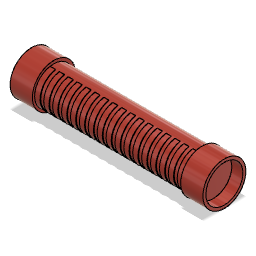
T-Stick (Autodesk Fusion 360 design; units mm, degrees)
Autodesk Fusion 360 part; units mm, degrees
note: some values were not read from the file. Chosen so that the rebuilt part matches the saved one: which bodies a step acts on.
sketch "Sketch1" plane through (0, 0, 0) normal (0, 0, 1) x (1, 0, 0)
  circle A0 centre (0, 0) radius 25
  circle A1 centre (0, 0) radius 29
  dimension "d3" = 50
  dimension "d4" = 4
  constraint coincident A0.centre A1.centre
  measures "d3" diameter of A0
extrude "Extrude1" add sketch "Sketch1" along normal blind 200 contours A0 makes body 1
extrude "Extrude2" add sketch "Sketch1" against normal blind 30 separate body makes body 2
extrude "Extrude3" add sketch "Sketch1" against normal blind 15 contours A0 bodies 1 2
sketch "Sketch2" plane through (0, 0, 200) normal (0, 0, 1) x (1, 0, 0)
  circle A0 centre (0, 0) radius 25
  circle A1 centre (0, 0) radius 29
  dimension "d9" = 4
extrude "Extrude4" add sketch "Sketch2" along normal blind 15 contours A0 bodies 1
extrude "Extrude5" add sketch "Sketch2" along normal blind 30 bodies 1
copy_body "CopyPasteBodies1" bodies 1 makes body 3
move_body "Move1" bodies 3 to x (1, 0, 0) y (0, 1, 0) z (0, 0, 1) at (0, 1, 0)
split "Split1" by plane through (0, 1, 200) normal (0, 0, -1) bodies 3 makes body 4 at (24.9689, -0.2461, 133.3333)
delete_body "RemoveBody1" bodies 3
split "Split2" by plane through (0, 1, 0) normal (0, 0, 1) bodies 4 makes body 5 at (24.9689, -0.2461, 133.3333)
delete_body "RemoveBody2" bodies 4
ref_plane "WorkPlane1" through (0, 26, 104.4776) normal (0, 1, 0) x (1, 0, 0)
sketch "Sketch3" plane through (0, 26, 104.4776) normal (0, 1, 0) x (1, 0, 0)
  line L0 (-26.9693, 97.1014) -> (24.8744, 97.1014)
  line L1 (24.8744, 97.1014) -> (24.8744, 92.1014)
  line L2 (24.8744, 92.1014) -> (-26.9693, 92.1014)
  line L3 (-26.9693, 92.1014) -> (-26.9693, 97.1014)
  line L4 (24.8744, 85.1014) -> (24.8744, 80.1014)
  line L5 (-26.9693, 80.1014) -> (-26.9693, 85.1014)
  line L6 (24.8744, 80.1014) -> (-26.9693, 80.1014)
  line L7 (-26.9693, 85.1014) -> (24.8744, 85.1014)
  line L8 (24.8744, 73.1014) -> (24.8744, 68.1014)
  line L9 (-26.9693, 68.1014) -> (-26.9693, 73.1014)
  line L10 (24.8744, 68.1014) -> (-26.9693, 68.1014)
  line L11 (-26.9693, 73.1014) -> (24.8744, 73.1014)
  line L12 (24.8744, 61.1014) -> (24.8744, 56.1014)
  line L13 (-26.9693, 56.1014) -> (-26.9693, 61.1014)
  line L14 (24.8744, 56.1014) -> (-26.9693, 56.1014)
  line L15 (-26.9693, 61.1014) -> (24.8744, 61.1014)
  line L16 (24.8744, 49.1014) -> (24.8744, 44.1014)
  line L17 (-26.9693, 44.1014) -> (-26.9693, 49.1014)
  line L18 (24.8744, 44.1014) -> (-26.9693, 44.1014)
  line L19 (-26.9693, 49.1014) -> (24.8744, 49.1014)
  line L20 (24.8744, 37.1014) -> (24.8744, 32.1014)
  line L21 (-26.9693, 32.1014) -> (-26.9693, 37.1014)
  line L22 (24.8744, 32.1014) -> (-26.9693, 32.1014)
  line L23 (-26.9693, 37.1014) -> (24.8744, 37.1014)
  line L24 (24.8744, 25.1014) -> (24.8744, 20.1014)
  line L25 (-26.9693, 20.1014) -> (-26.9693, 25.1014)
  line L26 (24.8744, 20.1014) -> (-26.9693, 20.1014)
  line L27 (-26.9693, 25.1014) -> (24.8744, 25.1014)
  line L28 (24.8744, 13.1014) -> (24.8744, 8.1014)
  line L29 (-26.9693, 8.1014) -> (-26.9693, 13.1014)
  line L30 (24.8744, 8.1014) -> (-26.9693, 8.1014)
  line L31 (-26.9693, 13.1014) -> (24.8744, 13.1014)
  line L32 (24.8744, 1.1014) -> (24.8744, -3.8986)
  line L33 (-26.9693, -3.8986) -> (-26.9693, 1.1014)
  line L34 (24.8744, -3.8986) -> (-26.9693, -3.8986)
  line L35 (-26.9693, 1.1014) -> (24.8744, 1.1014)
  line L36 (24.8744, -10.8986) -> (24.8744, -15.8986)
  line L37 (-26.9693, -15.8986) -> (-26.9693, -10.8986)
  line L38 (24.8744, -15.8986) -> (-26.9693, -15.8986)
  line L39 (-26.9693, -10.8986) -> (24.8744, -10.8986)
  line L40 (24.8744, -22.8986) -> (24.8744, -27.8986)
  line L41 (-26.9693, -27.8986) -> (-26.9693, -22.8986)
  line L42 (24.8744, -27.8986) -> (-26.9693, -27.8986)
  line L43 (-26.9693, -22.8986) -> (24.8744, -22.8986)
  line L44 (24.8744, -34.8986) -> (24.8744, -39.8986)
  line L45 (-26.9693, -39.8986) -> (-26.9693, -34.8986)
  line L46 (24.8744, -39.8986) -> (-26.9693, -39.8986)
  line L47 (-26.9693, -34.8986) -> (24.8744, -34.8986)
  line L48 (24.8744, -46.8986) -> (24.8744, -51.8986)
  line L49 (-26.9693, -51.8986) -> (-26.9693, -46.8986)
  line L50 (24.8744, -51.8986) -> (-26.9693, -51.8986)
  line L51 (-26.9693, -46.8986) -> (24.8744, -46.8986)
  line L52 (24.8744, -58.8986) -> (24.8744, -63.8986)
  line L53 (-26.9693, -63.8986) -> (-26.9693, -58.8986)
  line L54 (24.8744, -63.8986) -> (-26.9693, -63.8986)
  line L55 (-26.9693, -58.8986) -> (24.8744, -58.8986)
  line L56 (24.8744, -70.8986) -> (24.8744, -75.8986)
  line L57 (-26.9693, -75.8986) -> (-26.9693, -70.8986)
  line L58 (24.8744, -75.8986) -> (-26.9693, -75.8986)
  line L59 (-26.9693, -70.8986) -> (24.8744, -70.8986)
  line L60 (24.8744, -82.8986) -> (24.8744, -87.8986)
  line L61 (-26.9693, -87.8986) -> (-26.9693, -82.8986)
  line L62 (24.8744, -87.8986) -> (-26.9693, -87.8986)
  line L63 (-26.9693, -82.8986) -> (24.8744, -82.8986)
  dimension "d15" = 5
  dimension "d18" = 0
  dimension "d19" = -12
  constraint perpendicular L0 L1
  constraint parallel L0 L2
  constraint parallel L1 L3
  constraint horizontal L0
  measures "d15" distance of L0.start L2.end
extrude "Extrude6" cut sketch "Sketch3" against normal blind 90 bodies 5
box "BoxPrimitive1" cut length 211.5717 width 69.2223 height 5 placed x (0, 0, 1) y (1, 0, 0) z (0, 1, 0) at (-34.4543, 0, -6.8019) bodies 5 makes body 6 at (1.2482, 17.5528, 84.3761) makes body 7 at (1.2482, 17.5528, 60.3761) makes body 8 at (1.2482, 17.5528, 72.3761) makes body 9 at (1.2482, 17.5528, 48.3761) makes body 10 at (1.2482, 17.5528, 168.3761) makes body 11 at (1.2482, 17.5528, 120.3761) makes body 12 at (1.2482, 17.5528, 180.3761) makes body 13 at (1.2482, 17.5528, 96.3761) makes body 14 at (1.2482, 17.5528, 108.3761) makes body 15 at (1.2482, 17.5528, 24.3761) makes body 16 at (1.2482, 17.5528, 36.3761) makes body 17 at (1.2482, 17.5528, 144.3761) makes body 18 at (24.8525, -1.7121, 197.4587) makes body 19 at (1.2482, 17.5528, 156.3761) makes body 20 at (1.2482, 17.5528, 12.3761) makes body 21 at (4.1371, 10.9005, 7.3761) makes body 22 at (1.2482, 17.5528, 132.3761)
delete_body "RemoveBody3" bodies 18
combine "Combine1" operation add target body 1 tool bodies 19 17 5 16 8 21 12 15 6 10 14 22 11 13 20 9 7
move_body "Move2" bodies 1 to x (0, 1, 0) y (0, 0, 1) z (1, 0, 0) at (1, 0, -1)
